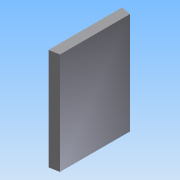
# Autodesk Inventor part: 10. Griff_Abdeckung
Saved by Autodesk Inventor 2011 SP1 (Build 150282100, 282)
## iProperties
Created: 2012-05-22
Part Number: 10. Griff_Abdeckung
Document SubType Name: Modeling
Designer: pburkhar
Density: 1 g/cm^3
Mass: 0.454759 g
Surface Area: 6.225 cm^2
Volume: 0.454759 cm^3
Author: pburkhar
Autodesk Inventor part; units mm, degrees
ref_plane "YZ Plane" through (0, 0, 0) normal (1, 0, 0) x (0, 1, 0)
ref_plane "XZ Plane" through (0, 0, 0) normal (0, 1, 0) x (-1, 0, 0)
ref_plane "XY Plane" through (0, 0, 0) normal (0, 0, 1) x (1, 0, 0)
sketch "Skizze1" plane through (0, 0, 0) normal (0, 0, 1) x (1, 0, 0)
  line L0 (11.3386, 6.1046) -> (9.5386, 6.422)
  line L1 (9.5386, 6.422) -> (9.5386, -7.2628)
  line L2 (9.5386, -7.2628) -> (11.3386, -6.9454)
  line L3 (11.3386, 6.1046) -> (9.5386, 6.422)
  line L4 (9.5386, 6.422) -> (9.5386, -7.2628)
  line L5 (9.5386, -7.2628) -> (11.3386, -6.9454)
  line L6 (11.3386, -6.9454) -> (11.3386, 6.1046)
  point P0 (0, 0)
  constraints: 14 end point, 2 collinear, 2 vertical
extrude "Extrusion1" add sketch "Skizze1" along normal blind 18.9
